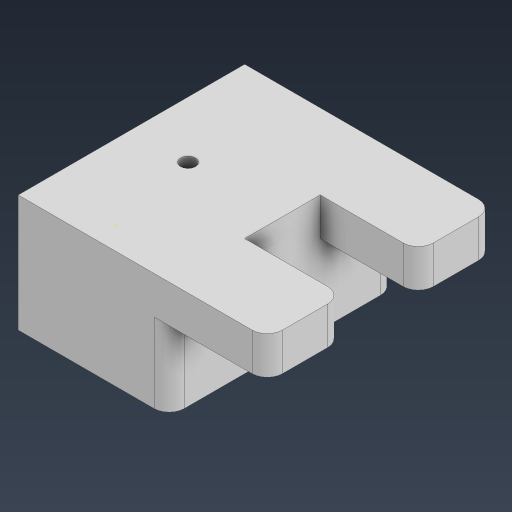
# Autodesk Inventor part: millenium_back_R
Saved by Autodesk Inventor 2024 (Build 280153000, 153)
## iProperties
Created: 2023-12-26
Part Number: millenium_back_R
Material: Generic
Document SubType Name: Modeling
Designer: Piter
Density: 1 g/cm^3
Appearance: Default
Author: Piter
Autodesk Inventor part; units mm, degrees
ref_plane "YZ Plane" through (0, 0, 0) normal (1, 0, 0) x (0, 1, 0)
ref_plane "XZ Plane" through (0, 0, 0) normal (0, 1, 0) x (-1, 0, 0)
ref_plane "XY Plane" through (0, 0, 0) normal (0, 0, 1) x (1, 0, 0)
sketch "Sketch1" plane through (0, 0, 0) normal (0, 1, 0) x (-1, 0, 0)
  line L0 (0, 0) -> (20, 0)
  line L1 (20, 0) -> (20, -30)
  line L2 (20, -30) -> (0, -30)
  line L3 (0, -30) -> (0, 0)
  dimension "d0" = 20
  dimension "d1" = 30
  constraints: 8 end point, 2 parallel, 1 horizontal, 1 perpendicular
  measures "d0" distance of L1.end L2.end
  measures "d1" distance of L0.end L1.end
extrude "Extrusion1" add sketch "Sketch1" along normal blind 17
sketch "Sketch2" plane through (0, 0, 0) normal (1, 0, 0) x (0, 0, -1)
  line L0 (30, 17) -> (0, 17) projected
  line L1 (0, 17) -> (10, 17)
  line L2 (10, 17) -> (10, 9)
  line L3 (10, 9) -> (0, 9)
  line L4 (0, 9) -> (0, 17)
  line L5 (10, 17) -> (20, 17)
  line L6 (20, 17) -> (30, 17)
  line L7 (30, 17) -> (30, 9)
  line L8 (30, 9) -> (20, 9)
  line L9 (20, 9) -> (20, 17)
  line L10 (10, 9) -> (20, 9)
  point P0 (0, 0)
  dimension "d4" = 10
  dimension "d5" = 8
  dimension "d6" = 10
  dimension "d7" = 10
  dimension "d8" = 8
  constraints: 20 end point, 4 parallel, 2 horizontal, 2 perpendicular, 1 point on line
  measures "d4" distance of L2.end L3.end
  measures "d5" distance of L1.end L2.end
  measures "d6" distance of L1.end L5.end
  measures "d7" distance of L7.end L8.end
  measures "d8" distance of L6.end L7.end
extrude "Extrusion2" add sketch "Sketch2" along normal blind 20 contours L7 L8 L9 L0 | L2 L3 L4 L0
sketch "Sketch3" plane through (0, 17, 0) normal (0, 1, 0) x (1, 0, 0)
  point P0 (0, 0)
extrude "Extrusion3" add sketch "Sketch2" along normal blind 7 contours L9 L10 L2 L0
move faces "Move1" translate (7, 0, 0) faces at (0, 3, -10)
move faces "Move2" translate (-3.25, 0, 0) faces at (-20, 11.3333, -20)
move faces "Move3" translate (5.25, 0, 0) faces at (-23.25, 11.3333, -20)
sketch "Sketch4" plane through (0, 17, 0) normal (0, 1, 0) x (1, 0, 0)
  line L0 (-18, 30) -> (-18, 0) projected
  line L1 (-18, 15) -> (7, 15)
  line L2 (7, 20) -> (7, 10) projected
  circle A0 centre (-5.5, 15) radius 1
  point P0 (0, 0)
  dimension "d22" = 2
  dimension "d28" = 12.5
  constraints: 3 midpoint, 2 end point, 1 centre point
  measures "d22" diameter of A0
  measures "d28" distance from line of L2 A0.centre
extrude "Extrusion4" cut sketch "Sketch4" against normal blind 12
fillet "Fillet1" radius 2 4 edges at (20, 13, 0) (20, 13, -30) (20, 13, -20) (20, 13, -10)
fillet "Fillet2" radius 2 2 edges at (7, 4.5, -30) (7, 4.5, 0)
move faces "Move4" translate (0, -1.5, 0) faces at (-9.6667, 0, -19.3333) (-10.3333, 8.6667, -30)
move faces "Move5" translate (5, 0, 0) faces at (-18, 10.8333, -20)
move faces "Move6" translate (0, -3, 0) faces at (4, 17, -3.3333) (-7, 8.1667, 0)
body "Solid1"
